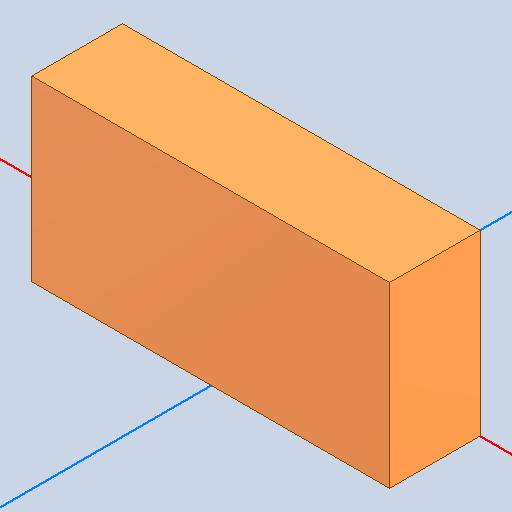
# Autodesk Inventor part: R0805
Saved by Autodesk Inventor 2022 (Build 260153000, 153)
## iProperties
Created: 2022-02-26
Part Number: R0805
Material: Типовые
Document SubType Name: Modeling
Designer: Petrov Ivan
Density: 1 g/cm^3
Appearance: R0805, R0805
Author: Petrov Ivan
Autodesk Inventor part; units mm, degrees
ref_plane "YZ Plane" through (0, 0, 0) normal (1, 0, 0) x (0, 1, 0)
ref_plane "XZ Plane" through (0, 0, 0) normal (0, 1, 0) x (-1, 0, 0)
ref_plane "XY Plane" through (0, 0, 0) normal (0, 0, 1) x (1, 0, 0)
sketch "R0805, R0805_21" plane through (0, 0, 0) normal (0, 0, 1) x (1, 0, 0)
  line L0 (-1.973, 0.983) -> (1.973, 0.983)
  line L1 (1.973, 0.983) -> (1.973, -0.983)
  line L2 (1.973, -0.983) -> (-1.973, -0.983)
  line L3 (-1.973, -0.983) -> (-1.973, 0.983)
  constraints: 8 end point
extrude "Выдавливание1" add sketch "R0805, R0805_21" along normal blind 1
